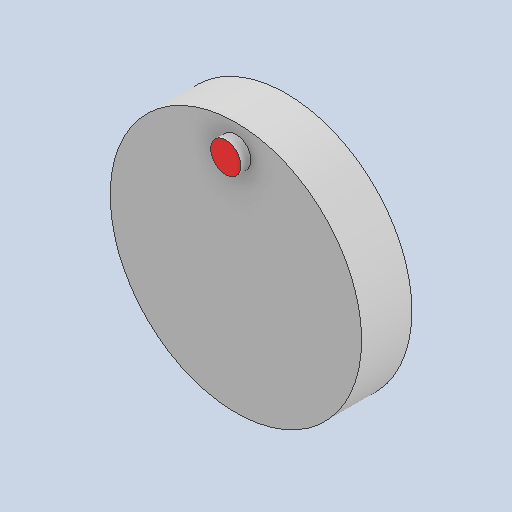
# Autodesk Inventor part: 원
Saved by Autodesk Inventor 2022 (Build 260153000, 153)
## iProperties
Created: 2022-10-28
Part Number: 원
Material: 일반
Document SubType Name: Modeling
Designer: whdls
Density: 1 g/cm^3
Appearance: 기본값
Author: whdls
Autodesk Inventor part; units mm, degrees
ref_plane "YZ Plane" through (0, 0, 0) normal (1, 0, 0) x (0, 1, 0)
ref_plane "XZ Plane" through (0, 0, 0) normal (0, 1, 0) x (-1, 0, 0)
ref_plane "XY Plane" through (0, 0, 0) normal (0, 0, 1) x (1, 0, 0)
sketch "스케치1" plane through (0, 0, 0) normal (0, 0, 1) x (1, 0, 0)
  circle A0 centre (0, 0) radius 12.5
  dimension "d0" = 25
  constraints: 1 centre point, 1 coincident
  measures "d0" diameter of A0
extrude "돌출1" add sketch "스케치1" along normal blind 5
sketch "스케치3" plane through (0, 0, 5) normal (0, 0, 1) x (1, 0, 0)
  circle A0 centre (0, 10) radius 1.5
  line L0 (-17.5, 0) -> (17.5, 0) construction
  line L1 (0, -17.5) -> (0, 17.5) construction
  point P0 (0, 0)
  dimension "d3" = 3
  dimension "d4" = 10
  constraints: 1 centre point, 1 point on line
  measures "d3" diameter of A0
  measures "d4" distance of point (0, 0) A0.centre
extrude "돌출2" add sketch "스케치3" along normal blind 1
